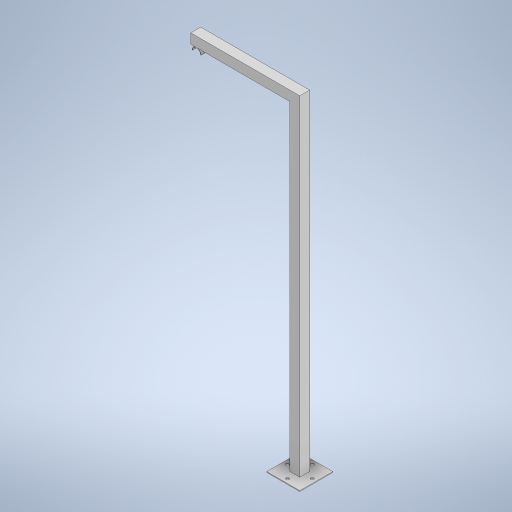
# Autodesk Inventor part: Sriel
Saved by Autodesk Inventor 2024 (Build 280153000, 153)
## iProperties
Created: 2023-04-22
Part Number: Sriel
Material: Genérico
Document SubType Name: Modeling
Designer: javie
Density: 1 g/cm^3
Appearance: Valor por defecto
Author: javie
Autodesk Inventor part; units mm, degrees
ref_plane "YZ Plane" through (0, 0, 0) normal (1, 0, 0) x (0, 1, 0)
ref_plane "XZ Plane" through (0, 0, 0) normal (0, 1, 0) x (-1, 0, 0)
ref_plane "XY Plane" through (0, 0, 0) normal (0, 0, 1) x (1, 0, 0)
sketch "Boceto1" plane through (0, 0, 0) normal (0, 1, 0) x (-1, 0, 0)
  line L0 (0, 0) -> (200, 0)
  line L1 (200, 0) -> (200, -200)
  line L2 (200, -200) -> (0, -200)
  line L3 (0, -200) -> (0, 0)
  dimension "d0" = 200
  dimension "d1" = 200
  constraints: 8 end point, 2 parallel, 1 horizontal, 1 perpendicular
  measures "d0" distance of L1.end L2.end
  measures "d1" distance of L0.end L1.end
extrude "Extrusión1" add sketch "Boceto1" along normal blind 5
sketch "Boceto2" plane through (0, 5, 0) normal (0, 1, 0) x (1, 0, 0)
  line L0 (-130, 70) -> (-70, 70)
  line L1 (-70, 70) -> (-70, 130)
  line L2 (-70, 130) -> (-130, 130)
  line L3 (-130, 130) -> (-130, 70)
  line L4 (-200, 200) -> (-200, 0) projected
  line L5 (-200, 0) -> (0, 0) projected
  point P0 (-130, 100)
  dimension "d4" = 60
  dimension "d5" = 60
  dimension "d6" = 70
  dimension "d7" = 70
  constraints: 8 end point, 2 parallel, 1 horizontal, 1 midpoint, 1 perpendicular
  measures "d4" distance of L2.end L1.end
  measures "d5" distance of L1.end L0.end
  measures "d6" distance from line of L4 point (-130, 100)
  measures "d7" distance between parallel lines of L5 L0
extrude "Extrusión2" add sketch "Boceto2" along normal blind 2000
sketch "Boceto3" plane through (-130, 5, -130) normal (-1, 0, 0) x (0, 0, 1)
  line L0 (0, 0) -> (0, 2000) projected
  line L1 (0, 2000) -> (60, 2000)
  line L2 (60, 2000) -> (60, 1940)
  line L3 (60, 1940) -> (0, 1940)
  line L4 (0, 1940) -> (0, 2000)
  point P0 (130, -5)
  dimension "d10" = 60
  dimension "d11" = 60
  constraints: 8 end point, 2 parallel, 1 horizontal, 1 perpendicular
  measures "d10" distance of L2.end L3.end
  measures "d11" distance of L1.end L2.end
extrude "Extrusión3" add sketch "Boceto3" along normal blind 600
sketch "Boceto4" plane through (-130, 5, -70) normal (0, 0, 1) x (1, 0, 0)
  arc A0 (-540, 1914) -> (-590, 1914) centre (-565, 1914) ccw
  line L0 (-600, 1940) -> (-600, 2000) projected
  line L1 (0, 1940) -> (-600, 1940) projected
  arc A1 (-537.5, 1914) -> (-592.5, 1914) centre (-565, 1914) ccw
  line L2 (-592.5, 1914) -> (-590, 1914)
  line L3 (-540, 1914) -> (-537.5, 1914)
  point P0 (130, -5)
  dimension "d14" = 50
  dimension "d15" = 35
  dimension "d16" = 26
  dimension "d17" = 55
  constraints: 4 end point, 4 point on circle, 2 centre point, 2 horizontal, 1 coincident
  measures "d14" diameter of A0
  measures "d15" distance from line of A0.centre L0
  measures "d16" distance from line of L1 A0.centre
  measures "d17" diameter of A1
extrude "Extrusión4" add sketch "Boceto4" against normal blind 60
sketch "Boceto5" plane through (0, 0, 0) normal (0, -1, 0) x (1, 0, 0)
  line L0 (0, 0) -> (0, -200) projected
  line L1 (0, -100) -> (-200, -100)
  line L2 (-200, -200) -> (-200, 0) projected
  line L3 (0, -200) -> (-200, -200) projected
  line L4 (-100, -200) -> (-100, 0)
  line L5 (-200, 0) -> (0, 0) projected
  circle A0 centre (-100, -175) radius 9.25
  circle A1 centre (-175, -100) radius 9.25
  circle A2 centre (-100, -25) radius 9.25
  circle A3 centre (-25, -100) radius 9.25
  point P0 (-100, -100)
  point P1 (-100, -100)
  point P2 (-100, -100)
  point P3 (-100, -100)
  dimension "d20" = 18.5
  dimension "d21" = 75
  dimension "d24" = 360
  constraints: 5 midpoint, 4 centre point, 4 end point, 2 coincident, 1 point on line, 11 other
  measures "d20" diameter of A0
  measures "d21" distance of point (-100, -100) A0.centre
extrude "Extrusión5" cut sketch "Boceto5" against normal blind 10 contours A3 L1 | L1 A3 | A2 L4 | L4 A2 | A0 L4 | L4 A0 | A1 L1 | L1 A1
